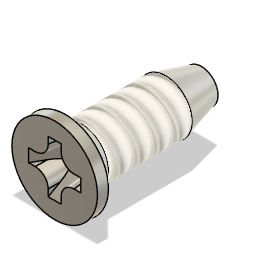
ca2e4d9a-e5a0-4fb4-92a4-221204bb6344 (Autodesk Fusion 360 design; units mm, degrees)
description: Parafuso Philips de cabeça chata escareada Tipo I ANSI B18.6.5M 2.2x0.8 x 6 Tipo B
part number: CRFCHTS ANSI B18.6.5M - 2.2 x 0.8 x 6 - B - I Aço grau 2 Liso
Autodesk Fusion 360 part; units mm, degrees
sketch "Sketch1" plane through (0, 0, 0) normal (0, 1, 0) x (1, 0, 0)
  line L0 (0, -2.2) -> (-1.75, -2.2)
  line L1 (-1.75, -2.2) -> (-1.75, -1.75)
  line L2 (-1.75, -1.75) -> (-1.1, -1.1)
  line L3 (-1.1, -1.1) -> (-1.1, 3.8)
  line L4 (-1.1, 3.8) -> (0, 3.8)
  line L5 (0, 3.8) -> (0, -2.2)
  dimension "d9" = 2.2
  dimension "d11" = 3.5
  dimension "d68" = 1.1
  dimension "d90" = 6
  dimension "d95" = 45
  constraint perpendicular L0 L1
  constraint vertical L3
  constraint perpendicular L3 L4
  constraint perpendicular L0 L5
  constraint collinear origin L0.start L4.end
  constraint horizontal L0
  constraint coincident origin L2
  measures "d68" distance of L0 L2.end
  measures "d90" distance of L0.start L4
  measures "d95" angle of L2 L5
revolve "Revolve1" add sketch "Sketch1" angle 360 about axis through (0, 0, -3.8) along (0, 0, 1) makes body 1
sketch "Sketch2" plane through (0, 0, 2.2) normal (0, 0, 1) x (1, 0, 0)
  line L0 (-0.265, 0.265) -> (-1.07, 0.265)
  line L1 (-1.07, 0.265) -> (-1.07, -0.265)
  line L2 (-1.07, -0.265) -> (-0.265, -0.265)
  line L3 (-0.265, -0.265) -> (-0.265, -1.07)
  line L4 (-0.265, -1.07) -> (0.265, -1.07)
  line L5 (0.265, -1.07) -> (0.265, -0.265)
  line L6 (0.265, -0.265) -> (1.07, -0.265)
  line L7 (1.07, -0.265) -> (1.07, 0.265)
  line L8 (1.07, 0.265) -> (0.265, 0.265)
  line L9 (0.265, 0.265) -> (0.265, 1.07)
  line L10 (0.265, 1.07) -> (-0.265, 1.07)
  line L11 (-0.265, 1.07) -> (-0.265, 0.265)
  dimension "d86" = 360
  dimension "d92" = 2.14
  dimension "d96" = 0.53
  constraint perpendicular L0 L1
  constraint horizontal L2
  constraint vertical L0.start L2.end
  constraint coincident L0.start L11.end
  measures "d92" distance of L4 L10
  measures "d96" distance of L0 L2
extrude "Extrude1" add sketch "Sketch2" against normal blind 1.54 draft -4 separate body makes body 2
draft "Draft1" angle -30 neutral plane through (0, 0, 2.2) pull (0, 0, 1) 4 faces at (-0.0524, 1.0341, 1.6867) (1.0341, 0.0524, 1.6867) (0.0524, -1.0341, 1.6867) (-1.0341, -0.0524, 1.6867) on bodies 2
fillet "Fillet3" radius 0.53 4 edges at (0.2112, 0.2112, 1.43) (-0.2112, 0.2112, 1.43) (-0.2112, -0.2112, 1.43) (0.2112, -0.2112, 1.43) on bodies 2
combine "Combine1" operation cut target body 1 tool bodies 2
thread "Thread1" "Metric Forming Screw Threads 2.2 2.2x0.8 2.2x0.8 6g" major diameter 2.17 minor diameter 1.575 pitch 0.8 angle 60 resizes the face on face at (-1.0986, 0.0548, -0.5333) on bodies 1
sketch "Sketch5" plane through (0, 0, 0) normal (0, 1, 0) x (1, 0, 0)
  line L0 (-1.122, 3.8) -> (-1.122, 2.2)
  line L1 (-1.122, 2.2) -> (-0.685, 3.8)
  line L2 (0, 3.8) -> (0, -2.2)
  line L3 (0, 3.8) -> (-1.122, 3.8)
  dimension "d75" = 1.122
  dimension "d93" = 0.685
  dimension "d94" = 1.6
  constraint vertical L0
  constraint coincident L2.start L3.start
  constraint perpendicular L0 L3
  constraint coincident L1.end L3
  measures "d75" distance of origin L0
  measures "d93" distance of L1.end L2
  measures "d94" distance of L0.end L3
revolve "Revolve2" cut sketch "Sketch5" angle 360 about axis through (0, 0, -3.8) along (0, 0, 1) bodies 1
equation "d9 = adsk_nomdia"
equation "d11 = adsk_headdia"
equation "adsk_nomlen = 6.00 mm"
equation "adsk_headh = 1.10 mm"
equation "adsk_headdia = 3.50 mm"
equation "adsk_nomdia = 2.20 mm"
equation "adsk_headang = 90.00 deg"
equation "adsk_phildia = 2.14 mm"
equation "d31 = -adsk_phildepth"
equation "adsk_philwidth = 0.53 mm"
equation "adsk_phildepth = 1.54 mm"
equation "adsk_startlen = 1.60 mm"
equation "d68 = adsk_headh"
equation "adsk_endpointdia = 1.37 mm"
equation "d75 = adsk_nomdia * 0.51"
equation "d80 = ( adsk_nomdia * 0.5 ) * tan(90 deg - adsk_headang * 0.5) + adsk_headh"
equation "d89 = adsk_philwidth"
equation "d90 = adsk_nomlen"
equation "d92 = adsk_phildia"
equation "d93 = adsk_endpointdia / 2"
equation "d94 = adsk_startlen"
equation "d95 = adsk_headang * 0.5"
equation "d96 = adsk_philwidth"
